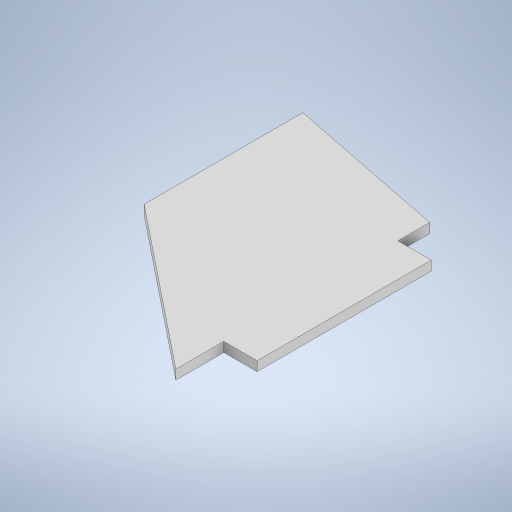
# Autodesk Inventor part: Stateczniki
Saved by Autodesk Inventor 2023.2 (Build 272271000, 271)
## iProperties
Created: 2022-12-18
Part Number: Stateczniki
Material: Generic
Document SubType Name: Modeling
Designer: Admin
Density: 1 g/cm^3
Appearance: Default
Author: Admin
Autodesk Inventor part; units mm, degrees
ref_plane "YZ Plane" through (0, 0, 0) normal (1, 0, 0) x (0, 1, 0)
ref_plane "XZ Plane" through (0, 0, 0) normal (0, 1, 0) x (-1, 0, 0)
ref_plane "XY Plane" through (0, 0, 0) normal (0, 0, 1) x (1, 0, 0)
sketch "Sketch1" plane through (0, 0, 0) normal (0, 1, 0) x (-1, 0, 0)
  line L0 (0, 0) -> (0, -80)
  line L1 (50, -90) -> (0, -80)
  line L2 (0, -70) -> (-10.5, -70)
  line L3 (-10.5, -70) -> (-10.5, -15.1)
  line L4 (-10.5, -15.1) -> (0, -15.1)
  line L5 (0, -15.1) -> (-4, -15.1)
  line L6 (-4, -15.1) -> (-4, -70) construction
  line L7 (50, -90) -> (50, -40)
  line L8 (50, -40) -> (0, 0)
  dimension "d0" = 80
  dimension "d1" = 50
  dimension "d5" = 10
  dimension "d6" = 54.9
  dimension "d9" = 4
  constraints: 18 end point, 4 point on line, 3 perpendicular, 2 vertical, 1 horizontal
  measures "d0" distance of L0.start L0.end
  measures "d1" horizontal distance of L0.end L1.start
  measures "d5" vertical distance of L0.end L2.end
  measures "d6" distance of L2.end L3.end
  measures "d9" distance of L4.end L5.end
extrude "Extrusion1" add sketch "Sketch1" along normal mid plane 3
body "Solid1"
